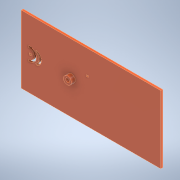
# Autodesk Inventor part: Lid
Saved by Autodesk Inventor 2022.2 (Build 262287010, 287A)
## iProperties
Created: 2022-03-17
Part Number: Lid
Material: Genérico
Document SubType Name: Modeling
Designer: mabel
Density: 1 g/cm^3
Appearance: Suave - Naranja claro
Author: mabel
Autodesk Inventor part; units mm, degrees
ref_plane "YZ Plane" through (0, 0, 0) normal (1, 0, 0) x (0, 1, 0)
ref_plane "XZ Plane" through (0, 0, 0) normal (0, 1, 0) x (-1, 0, 0)
sketch "Boceto2" plane through (0, 0, 0) normal (0, 0, 1) x (1, 0, 0)
  line L0 (130, -85) -> (-130, -85)
  line L1 (-130, -85) -> (-130, 85)
  line L2 (-130, 85) -> (130, 85)
  line L3 (130, 85) -> (130, -85)
  line L4 (130, -85) -> (-130, 85) construction
  line L5 (-130, -85) -> (130, 85) construction
  point P0 (0, 0)
  dimension "d0" = 260
  dimension "d1" = 170
  constraints: 12 end point, 2 midpoint, 2 parallel, 1 horizontal, 1 perpendicular
  measures "d0" distance of L1.end L2.end
  measures "d1" distance of L0.end L1.end
extrude "Extrusión1" add sketch "Boceto2" along normal blind 5
sketch "Boceto3" plane through (0, 0, 5) normal (0, 0, 1) x (1, 0, 0)
  line L0 (-95, 0) -> (-4.19, 0) construction
  circle A0 centre (-95, 0) radius 2.625
  circle A1 centre (-4.19, 0) radius 9.875
  line L1 (-130, 85) -> (-130, -85) projected
  line L2 (130, -85) -> (130, 85) projected
  line L3 (-130, -85) -> (130, -85) projected
  line L4 (130, 0) -> (80, 0) construction
  line L5 (80, 0) -> (80, -23.2237) construction
  arc A2 (-110, -17.625) -> (-110, 17.625) centre (-110, 0) ccw
  arc A3 (-110, -12.375) -> (-110, 12.375) centre (-110, 0) ccw
  arc A4 (-110, 17.625) -> (-110, 12.375) centre (-110, 15) ccw
  arc A5 (-110, -12.375) -> (-110, -17.625) centre (-110, -15) ccw
  point P0 (0, 0)
  point P1 (-130, 0)
  point P2 (-92.375, 0)
  point P3 (-97.625, 0)
  dimension "d7" = 5.25
  dimension "d8" = 19.75
  dimension "d14" = 85
  dimension "d29" = 50
  dimension "d31" = 35
  dimension "d32" = 134.19
  constraints: 8 point on circle, 6 centre point, 6 end point, 3 coincident, 2 horizontal, 2 midpoint, 1 perpendicular
  measures "d7" diameter of A0
  measures "d8" diameter of A1
  measures "d14" distance from line of L3 L0.end
  measures "d29" distance of L4.start L4.end
  measures "d31" distance from line of A0.centre L1
  measures "d32" distance from line of L2 A1.centre
sketch "Boceto5" plane through (0, 0, 0) normal (0, 0, -1) x (-1, 0, 0)
  line L0 (-130, -85) -> (-130, 85) projected
  line L1 (130, -85) -> (-130, -85)
  line L2 (-130, -85) -> (-130, 85)
  line L3 (-130, 85) -> (130, 85)
  line L4 (130, 85) -> (130, -85)
  line L5 (130, -85) -> (-130, 85) construction
  line L6 (-130, -85) -> (130, 85) construction
  line L7 (119.5, 74.5) -> (-119.5, 74.5)
  line L8 (-119.5, 74.5) -> (-119.5, -74.5)
  line L9 (-119.5, -74.5) -> (119.5, -74.5)
  line L10 (119.5, -74.5) -> (119.5, 74.5)
  circle A0 centre (95, 0) radius 2.625 projected
  circle A1 centre (95, 0) radius 2.625
  point P0 (0, 0)
  dimension "d23" = 10.5
  dimension "d25" = 5.25
  constraints: 20 end point, 4 parallel, 2 midpoint, 2 perpendicular, 1 centre point, 1 coincident, 1 horizontal, 3 other
  measures "d23" distance between parallel lines of L3 L7
  measures "d25" diameter of A1
extrude "Extrusión4" [suppressed]
sketch "Boceto6" plane through (0, 0, 5) normal (0, 0, 1) x (1, 0, 0)
  circle A0 centre (-4.19, 0) radius 10.125 projected
  line L0 (-4.19, 0) -> (35.81, 0)
  line L1 (35.81, 0) -> (35.81, 25)
  line L2 (37.81, 23.5) -> (33.81, 23.5)
  line L3 (33.81, 23.5) -> (33.81, 26.5)
  line L4 (33.81, 26.5) -> (37.81, 26.5)
  line L5 (37.81, 26.5) -> (37.81, 23.5)
  line L6 (37.81, 23.5) -> (33.81, 26.5) construction
  line L7 (33.81, 23.5) -> (37.81, 26.5) construction
  point P0 (0, 0)
  dimension "d35" = 40
  dimension "d36" = 25
  dimension "d38" = 4
  dimension "d39" = 3
  constraints: 16 end point, 2 horizontal, 2 midpoint, 2 parallel, 2 perpendicular
  measures "d35" distance of L0.start L0.end
  measures "d36" distance of L0.end L1.end
  measures "d38" distance of L3.end L4.end
  measures "d39" distance of L2.end L3.end
extrude "Extrusión5" cut sketch "Boceto6" against normal blind 1.4 contours L2 L3 L4 L5
sketch "Boceto8" plane through (0, 0, 5) normal (0, 0, 1) x (1, 0, 0)
  line L0 (33.81, 23.5) -> (33.81, 26.5) projected
  line L1 (33.81, 23.5) -> (37.81, 23.5)
  line L2 (37.81, 23.5) -> (37.81, 22.5)
  line L3 (37.81, 22.5) -> (33.81, 22.5)
  line L4 (33.81, 22.5) -> (33.81, 23.5)
  point P0 (0, 0)
  dimension "d42" = 4
  dimension "d43" = 1
  constraints: 8 end point, 2 parallel, 1 horizontal, 1 perpendicular
  measures "d42" distance of L2.end L3.end
  measures "d43" distance of L1.end L2.end
extrude "Extrusión6" cut sketch "Boceto8" against normal through all
sketch "Boceto10" plane through (0, 0, -4) normal (0, 0, -1) x (-1, 0, 0)
  circle A0 centre (95, 0) radius 2.625 projected
  circle A1 centre (95, 0) radius 7.5
  point P0 (0, 0)
  dimension "d51" = 15
  constraints: 1 centre point, 1 coincident
  measures "d51" diameter of A1
ref_plane "Plano de trabajo1" through (-95, 0, 0) normal (0, 0, -1) x (-1, 0, 0)
sketch "Boceto12" plane through (0, 0, 5) normal (0, 0, 1) x (1, 0, 0)
  circle A0 centre (-95, 0) radius 2.625 construction
  circle A1 centre (-95, 0) radius 18.5 construction
  circle A2 centre (-95, 0) radius 20 construction
  circle A3 centre (-95, 0) radius 7.5 construction
  line L0 (-95, 0) -> (-82.5, 0) construction
  circle A4 centre (-82.5, 0) radius 3
  line L1 (-95, 0) -> (-107.5, 0) construction
  circle A5 centre (-107.5, 0) radius 3
  circle A6 centre (-107.5, 0) radius 1.5 construction
  circle A7 centre (-82.5, 0) radius 1.5 construction
  line L2 (-82.5, 0) -> (-97.5, 0) construction
  line L3 (-97.5, 0) -> (-97.5, 18.5) construction
  arc A8 (-89.1168, -15.9286) -> (-89.9998, 16.363) centre (-97.5, 0) ccw
  arc A9 (-91.9112, -10.6191) -> (-92.6345, 10.9694) centre (-97.5, 0) ccw
  arc A10 (-91.9112, -10.6191) -> (-89.1168, -15.9286) centre (-90.514, -13.2739) ccw
  arc A11 (-89.9998, 16.363) -> (-92.6345, 10.9694) centre (-91.2508, 13.6338) ccw
  arc A12 (-91.9112, -10.6191) -> (-89.1168, -15.9286) centre (-90.514, -13.2739) ccw
  arc A13 (-92.595, 10.9517) -> (-92.4052, 10.8647) centre (-91.2508, 13.6338) ccw
  arc A14 (-91.9112, -10.6191) -> (-89.1168, -15.9286) centre (-90.514, -13.2739) ccw
  arc A15 (-89.8154, -14.6013) -> (-90.6248, 14.9994) centre (-97.5, 0) ccw
  arc A16 (-90.6248, 14.9994) -> (-91.9757, 12.318) centre (-91.2508, 13.6338) ccw
  arc A17 (-91.2126, -11.9465) -> (-91.9757, 12.318) centre (-97.5, 0) ccw
  arc A18 (-91.2126, -11.9465) -> (-89.8154, -14.6013) centre (-90.514, -13.2739) ccw
  circle A19 centre (-82.5, 0) radius 1.5
  line L4 (-130, 85) -> (-130, -85) projected
  line L5 (-130, -85) -> (130, -85) projected
  point P0 (0, 0)
  point P1 (-89.8154, -14.6013)
  point P2 (-91.2126, -11.9465)
  point P3 (-84.225, -2.4545)
  point P4 (-85.5, 0)
  point P5 (-79.5, 0)
  point P6 (-81.225, -2.7156)
  point P7 (-84.225, 2.4545)
  point P8 (-81.225, 2.7156)
  point P9 (-84, 0)
  point P10 (-81, 0)
  dimension "d57" = 37
  dimension "d58" = 40
  dimension "d59" = 15
  dimension "d60" = 12.5
  dimension "d61" = 6
  dimension "d62" = 12.5
  dimension "d63" = 6
  dimension "d64" = 3
  dimension "d65" = 3
  dimension "d126" = 15
  dimension "d127" = 6
  dimension "d128" = 6
  dimension "d129" = 1.5
  dimension "d130" = 1.5
  dimension "d135" = 3
  dimension "d137" = 38.7492
  dimension "d138" = 98.6338
  constraints: 24 point on circle, 19 centre point, 12 coincident, 8 end point, 4 tangent, 2 horizontal, 1 point on line, 1 vertical, 2 other
  measures "d57" diameter of A1
  measures "d58" diameter of A2
  measures "d59" diameter of A3
  measures "d60" distance of L0.start L0.end
  measures "d61" diameter of A4
  measures "d62" distance of L0.start L1.end
  measures "d63" diameter of A5
  measures "d64" diameter of A6
  measures "d65" diameter of A7
  measures "d126" distance of L2.start L2.end
  measures "d127" diameter of A13
  measures "d128" diameter of A14
  measures "d129" radial gap between concentric circles of A8 A15
  measures "d130" radial gap between concentric circles of A14 A18
  measures "d135" diameter of A19
  measures "d137" distance from line of L4 A11.centre
  measures "d138" distance from line of L5 A11.centre
extrude "Extrusión10" cut sketch "Boceto12" against normal blind 1.5 contours A4 A15 | A15 A19 A17 A4 | A4 A17 A19 A15 | A17 A4 | A19 | A5
sketch "Boceto13" plane through (-82.5, 0, 3.5) normal (0, 0, 1) x (1, 0, 0)
  circle A0 centre (0, 0) radius 1.5
  circle A1 centre (-25, 0) radius 3 projected
  circle A2 centre (-25, 0) radius 1.5
  point P0 (82.5, 0)
  dimension "d68" = 3
  dimension "d69" = 3
  constraints: 2 centre point, 1 coincident
  measures "d68" diameter of A0
  measures "d69" diameter of A2
extrude "Extrusión11" cut sketch "Boceto13" against normal through all contours A0 | A2
extrude "Extrusión12" [suppressed]
extrude "Extrusión13" add sketch "Boceto3" along normal blind 10 contours A1
sketch "Boceto15" plane through (-4.19, 0, 15) normal (0, 0, 1) x (1, 0, 0)
  circle A0 centre (0, 0) radius 5
  circle A1 centre (0, 0) radius 74 construction
  circle A2 centre (-90.81, 0) radius 2.625 construction
  circle A3 centre (-90.81, 0) radius 20 construction
  point P0 (4.19, 0)
  dimension "d77" = 10
  dimension "d80" = 148
  dimension "d82" = 40
  constraints: 3 centre point, 2 coincident
  measures "d77" diameter of A0
  measures "d80" diameter of A1
  measures "d82" diameter of A3
extrude "Extrusión14" cut sketch "Boceto15" against normal through all
sketch "Boceto16" plane through (0, 0, -4) normal (0, 0, -1) x (-1, 0, 0)
  line L0 (119.5, 74.5) -> (-119.5, 74.5) projected
  line L1 (-119.5, 74.5) -> (119.5, 74.5)
  line L2 (119.5, 74.5) -> (119.5, -74.5)
  line L3 (119.5, -74.5) -> (-119.5, -74.5)
  line L4 (-119.5, -74.5) -> (-119.5, 74.5)
  line L5 (-114.5, 69.5) -> (114.5, 69.5)
  line L6 (114.5, 69.5) -> (114.5, -69.5)
  line L7 (114.5, -69.5) -> (-114.5, -69.5)
  line L8 (-114.5, -69.5) -> (-114.5, 69.5)
  point P0 (0, 0)
  dimension "d83" = 5
  constraints: 16 end point, 4 parallel, 2 perpendicular, 1 horizontal, 3 other
  measures "d83" distance between parallel lines of L4 L8
extrude "Extrusión15" [suppressed]
sketch "Boceto17" plane through (0, 0, 5) normal (0, 0, 1) x (1, 0, 0)
  circle A0 centre (-95, 0) radius 2.625 construction
  circle A1 centre (-4.19, 0) radius 5 construction
  circle A2 centre (-4.19, 0) radius 40
  circle A3 centre (-4.19, 0) radius 15
  point P0 (0, 0)
  dimension "d87" = 80
  dimension "d88" = 30
  constraints: 2 centre point, 2 coincident
  measures "d87" diameter of A2
  measures "d88" diameter of A3
sketch "Boceto20" plane through (0, 0, 5) normal (0, 0, 1) x (1, 0, 0)
  line L0 (130, 85) -> (-130, 85) projected
  line L1 (130, -85) -> (130, 85)
  line L2 (130, 85) -> (220, 85)
  line L3 (220, 85) -> (220, -85)
  line L4 (220, -85) -> (130, -85)
  line L5 (130, -85) -> (130, 85)
  point P0 (0, 0)
  dimension "d115" = 90
  constraints: 10 end point, 2 parallel, 1 horizontal, 1 perpendicular
  measures "d115" distance of L3.end L4.end
extrude "Extrusión22" add sketch "Boceto20" against normal blind 5
extrude "Extrusión23" cut sketch "Boceto3" against normal through all contours A0
extrude "Extrusión24" cut sketch "Boceto3" against normal blind 5 contours A2 A5 A3 A0 | A0 A3 A4 A2
extrude "Extrusión25" cut sketch "Boceto12" against normal blind 1.5 contours A8 A10 A9 A4 A17 A18 A15 | A4 A15 A16 A17 A9 A11 A8
extrude "Extrusión26" cut sketch "Boceto12" against normal through all contours A15 A19 A17 A4 | A4 A17 A16 A15 | A15 A18 A17 A4 | A4 A17 A19 A15
